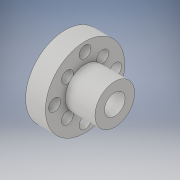
# Autodesk Inventor part: WheelandSprocketComboHub
Saved by Autodesk Inventor 2017 (Build 210142000, 142)
## iProperties
Created: 2018-04-04
Part Number: WheelandSprocketComboHub
Material: Generic
Document SubType Name: Modeling
Designer: User
Density: 1 g/cm^3
Appearance: Default
Author: User
Autodesk Inventor part; units mm, degrees
ref_plane "YZ Plane" through (0, 0, 0) normal (1, 0, 0) x (0, 1, 0)
ref_plane "XZ Plane" through (0, 0, 0) normal (0, 1, 0) x (-1, 0, 0)
ref_plane "XY Plane" through (0, 0, 0) normal (0, 0, 1) x (1, 0, 0)
sketch "Sketch1" plane through (0, 0, 0) normal (1, 0, 0) x (0, 1, 0)
  circle A0 centre (0, 0) radius 12.7
  circle A1 centre (9.779, 0) radius 1.905
  circle A2 centre (5.6576, -5.6576) radius 1.905
  line L0 (5.6576, -5.6576) -> (0, 0)
  line L1 (0, 0.0631) -> (0, -4.7425)
  circle A3 centre (0, 9.779) radius 1.905
  circle A4 centre (-9.779, 0) radius 1.905
  circle A5 centre (0, -9.779) radius 1.905
  circle A6 centre (5.6576, 5.6576) radius 1.905
  circle A7 centre (-5.6576, 5.6576) radius 1.905
  circle A8 centre (-5.6576, -5.6576) radius 1.905
  circle A9 centre (0, 0) radius 3.302
  dimension "d0" = 25.4
  dimension "d1" = 3.81
  dimension "d2" = 3.81
  dimension "d3" = 9.779
  dimension "d6" = 45
  dimension "d9" = 360
  dimension "d13" = 360
  dimension "d15" = 6.604
  constraints: 10 centre point, 4 end point, 2 coincident, 2 point on line, 1 vertical, 18 other
  measures "d0" diameter of A0
  measures "d1" diameter of A1
  measures "d2" diameter of A2
  measures "d3" distance of point (0, 0) A1.centre
  measures "d6" angle of L1 L0
  measures "d15" diameter of A9
extrude "Extrusion1" add sketch "Sketch1" along normal blind 6.35
sketch "Sketch2" plane through (6.35, 0, 0) normal (1, 0, 0) x (0, 0, -1)
  circle A0 centre (0, 0) radius 3.302 projected
  circle A1 centre (0, 0) radius 6.35
  point P0 (0, 0)
  dimension "d18" = 12.7
  constraints: 1 centre point, 1 coincident
  measures "d18" diameter of A1
extrude "Extrusion2" add sketch "Sketch2" along normal blind 9.525
body "Solid1"
